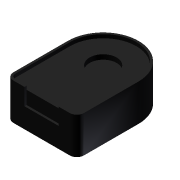
# Autodesk Inventor part: HEDS-5500_B
Saved by Autodesk Inventor 2011 SP1 (Build 150282100, 282)
## iProperties
Created: 2012-12-12
Part Number: HEDS-5500_B
Document SubType Name: Modeling
Designer: arihon
Density: 1 g/cm^3
Author: arihon
Autodesk Inventor part; units mm, degrees
ref_plane "YZ Plane" through (0, 0, 0) normal (1, 0, 0) x (0, 1, 0)
ref_plane "XZ Plane" through (0, 0, 0) normal (0, 1, 0) x (-1, 0, 0)
ref_plane "XY Plane" through (0, 0, 0) normal (0, 0, 1) x (1, 0, 0)
sketch "スケッチ1" plane through (0, 0, 0) normal (0, 0, 1) x (1, 0, 0)
  line L0 (-15, 0) -> (15, 0)
  line L1 (15, 0) -> (15, -26.2)
  line L2 (15, -26.2) -> (-15, -26.2)
  line L3 (-15, -26.2) -> (-15, 0)
  circle A0 centre (0, 0) radius 15
  dimension "d0" = 30
  dimension "d1" = 15
  dimension "d2" = 26.2
  dimension "d3" = 0
  constraints: 8 end point, 2 parallel, 1 coincident, 1 horizontal, 1 horizontal alignment, 1 perpendicular, 2 other
  measures "d0" distance of L1.end L2.end
  measures "d1" distance from line of L3 point (0, 0)
  measures "d2" distance of L2.end L0.start
  measures "d3" distance from line of point (0, 0) L0
extrude "押し出し1" add sketch "スケッチ1" along normal blind 15.6
sketch "スケッチ2" plane through (0, 0, 15.6) normal (0, 0, 1) x (1, 0, 0)
  arc A0 (15, 0) -> (-15, 0) centre (0, 0) ccw projected
  line L0 (-15, -26.2) -> (-15, 0) projected
  line L1 (15, -26.2) -> (-15, -26.2) projected
  line L2 (15, 0) -> (15, -26.2) projected
  line L3 (-14.1, 0) -> (14.1, 0)
  line L4 (14.1, 0) -> (14.1, -25.3)
  line L5 (14.1, -25.3) -> (-14.1, -25.3)
  line L6 (-14.1, -25.3) -> (-14.1, 0)
  circle A1 centre (0, 0) radius 14.1
  dimension "d6" = 0.9
  dimension "d7" = 0.9
  dimension "d8" = 0.9
  constraints: 8 end point, 2 parallel, 1 coincident, 1 horizontal, 1 horizontal alignment, 1 perpendicular, 2 other
  measures "d6" distance between parallel lines of L0 L6
  measures "d7" distance between parallel lines of L2 L4
  measures "d8" distance between parallel lines of L1 L5
extrude "押し出し2" cut sketch "スケッチ2" against normal blind 1.5 contours A1 L3 | A1 L4 L5 L6 | L3 A1
sketch "スケッチ3" plane through (0, 0, 14.1) normal (0, 0, 1) x (1, 0, 0)
  arc A0 (14.1, 0) -> (-14.1, 0) centre (0, 0) ccw projected
  circle A1 centre (0, 0) radius 5.75
  dimension "d11" = 11.5
  constraints: 1 centre point, 1 coincident
  measures "d11" diameter of A1
extrude "押し出し3" cut sketch "スケッチ3" against normal blind 2
fillet "フィレット1" radius 3 2 edges at (15, -26.2, 7.8) (-15, -26.2, 7.8)
fillet "フィレット2" radius 2.1 2 edges at (-14.1, -25.3, 14.85) (14.1, -25.3, 14.85)
sketch "スケッチ4" plane through (0, 0, 15.6) normal (0, 0, 1) x (1, 0, 0)
  line L0 (12, -26.2) -> (-12, -26.2) projected
  arc A0 (15, 0) -> (-15, 0) centre (0, 0) ccw projected
  line L1 (-12, -25.3) -> (12, -25.3) projected
  line L2 (-7.25, -25.3) -> (7.25, -25.3)
  line L3 (7.25, -25.3) -> (7.25, -26.2)
  line L4 (7.25, -26.2) -> (-7.25, -26.2)
  line L5 (-7.25, -26.2) -> (-7.25, -25.3)
  dimension "d16" = 14.5
  dimension "d17" = 7.25
  constraints: 8 end point, 2 parallel, 2 point on line, 1 horizontal, 1 perpendicular
  measures "d16" distance between parallel lines of L5 L3
  measures "d17" distance from line of L5 A0.centre
extrude "押し出し4" cut sketch "スケッチ4" against normal blind 7.1
equation "\"d1\" = 0.5 * d0"
equation "\"d7\" = d6"
equation "\"d8\" = d6"
equation "\"d17\" = 0.5 * d16"
